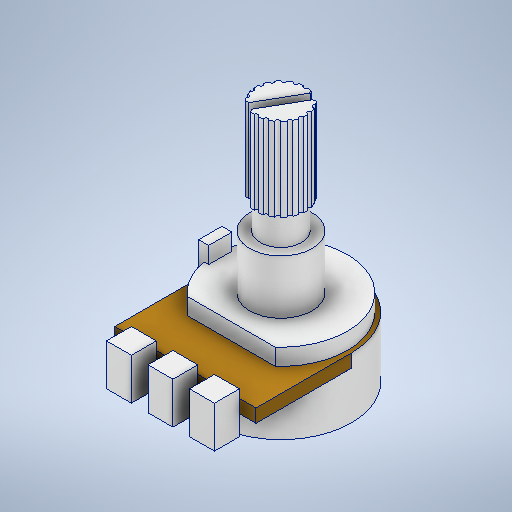
# Autodesk Inventor part: volume
Saved by Autodesk Inventor 2026.1 (Build 301233020, 233B)
## iProperties
Created: 2026-02-01
Part Number: volume
Material: アルミニウム 6061
Document SubType Name: Modeling
Designer: hibik
Density: 2.7 g/cm^3
Appearance: アルミニウム - フラット
Author: hibik
Autodesk Inventor part; units mm, degrees
ref_plane "YZ Plane" through (0, 0, 0) normal (1, 0, 0) x (0, 1, 0)
ref_plane "XZ Plane" through (0, 0, 0) normal (0, 1, 0) x (-1, 0, 0)
ref_plane "XY Plane" through (0, 0, 0) normal (0, 0, 1) x (1, 0, 0)
sketch "スケッチ1" plane through (0, 0, 0) normal (0, 1, 0) x (-1, 0, 0)
  circle A0 centre (0, 0) radius 8.5
  dimension "d0" = 17
  constraints: 1 centre point, 1 coincident
  measures "d0" diameter of A0
extrude "押し出し1" add sketch "スケッチ1" along normal blind 9.3
sketch "スケッチ2" plane through (0, 9.3, 0) normal (0, 1, 0) x (1, 0, 0)
  circle A0 centre (0, 0) radius 3
  dimension "d3" = 6
  constraints: 1 centre point, 1 coincident
  measures "d3" diameter of A0
extrude "押し出し2" add sketch "スケッチ2" along normal blind 20
sketch "スケッチ3" plane through (0, 9.3, 0) normal (0, 1, 0) x (1, 0, 0)
  circle A0 centre (0, 0) radius 3.75
  dimension "d6" = 7.5
  constraints: 1 centre point, 1 coincident
  measures "d6" diameter of A0
extrude "押し出し3" add sketch "スケッチ3" along normal blind 6.5
sketch "スケッチ4" plane through (0, 15.8, 0) normal (0, 1, 0) x (1, 0, 0)
  circle A0 centre (0, 0) radius 3 projected
  circle A1 centre (0, 0) radius 2.5
  dimension "d9" = 5
  constraints: 1 centre point, 1 coincident
  measures "d9" diameter of A1
extrude "押し出し4" cut sketch "スケッチ4" along normal blind 3.5
sketch "スケッチ5" plane through (0, 9.3, 0) normal (0, 1, 0) x (1, 0, 0)
  circle A0 centre (0, 0) radius 6
  circle A1 centre (0, 0) radius 8.5 projected
  dimension "d12" = 12
  constraints: 1 centre point, 1 coincident
  measures "d12" diameter of A0
extrude "押し出し5" cut sketch "スケッチ5" against normal blind 2
sketch "スケッチ6" plane through (0, 7.3, 0) normal (0, 1, 0) x (1, 0, 0)
  circle A0 centre (0, 0) radius 8.5 projected
  line L0 (-8.5, 0) -> (8.5, 0)
  line L1 (8.5, 0) -> (8.5, -11.5)
  line L2 (8.5, -11.5) -> (-8.5, -11.5)
  line L3 (-8.5, -11.5) -> (-8.5, 0)
  dimension "d15" = 11.5
  constraints: 8 end point, 2 parallel, 2 vertical, 1 horizontal, 1 perpendicular, 2 other
  measures "d15" distance of L2.end L0.start
extrude "押し出し6" add sketch "スケッチ6" against normal blind 1.6 contours L1 L2 L3 A0
sketch "スケッチ7" plane through (-8.5, 7.3, 11.5) normal (0, 0, 1) x (1, 0, 0)
  line L0 (7, 1) -> (10, 1)
  line L1 (10, 1) -> (10, -4)
  line L2 (10, -4) -> (7, -4)
  line L3 (7, -4) -> (7, 1)
  line L4 (0, 0) -> (17, 0) projected
  point P0 (8.5, -7.3)
  point P1 (8.5, -4)
  point P2 (8.5, 1)
  dimension "d18" = 5
  dimension "d19" = 3
  dimension "d20" = 1
  constraints: 8 end point, 2 midpoint, 2 parallel, 1 horizontal, 1 perpendicular, 1 vertical alignment
  measures "d18" distance of L0.end L1.end
  measures "d19" distance of L1.end L2.end
  measures "d20" distance from line of L4 point (8.5, 1)
extrude "押し出し7" add sketch "スケッチ7" along normal blind 3
pattern_linear "矩形状パターン1" count 2 spacing 5 along (1, 0, 0) count 2 spacing 5 along (-1, 0, 0) of "押し出し7"
sketch "スケッチ8" plane through (0, 7.3, 0) normal (0, 1, 0) x (1, 0, 0)
  line L0 (-8.5, -1.4) -> (-7.3, -1.4)
  line L1 (-7.3, -1.4) -> (-7.3, 1.4)
  line L2 (-7.3, 1.4) -> (-8.5, 1.4)
  line L3 (-8.5, 1.4) -> (-8.5, -1.4)
  point P0 (0, 0)
  point P1 (-8.5, 0)
  point P2 (-8.5, 0)
  dimension "d29" = 2.8
  dimension "d30" = 1.2
  constraints: 8 end point, 2 parallel, 1 coincident, 1 horizontal, 1 midpoint, 1 perpendicular
  measures "d29" distance of L2.end L0.start
  measures "d30" distance of L1.end L2.end
extrude "押し出し8" add sketch "スケッチ8" along normal blind 4
sketch "スケッチ9" plane through (0, 7.3, 0) normal (0, 1, 0) x (1, 0, 0)
  circle A0 centre (0, 0) radius 8
  line L0 (-5.2915, -6) -> (5.2915, -6)
  circle A1 centre (0, 0) radius 6 projected
  point P0 (0, -6)
  dimension "d33" = 16
  constraints: 2 end point, 2 point on circle, 1 centre point, 1 coincident, 1 horizontal, 1 tangent
  measures "d33" diameter of A0
extrude "押し出し9" add sketch "スケッチ9" along normal blind 2 contours A0 L0 picked at (7.1897, 1.149)
sketch "スケッチ10" plane through (0, 29.3, 0) normal (0, 1, 0) x (1, 0, 0)
  line L0 (-2.308, -2.9976) -> (-1.442, -3.4976)
  line L1 (-1.442, -3.4976) -> (2.308, 2.9976)
  line L2 (2.308, 2.9976) -> (1.442, 3.4976)
  line L3 (1.442, 3.4976) -> (-2.308, -2.9976)
  line L4 (-1.875, -3.2476) -> (1.875, 3.2476)
  line L5 (0, 20.6367) -> (0, -20.3561) construction
  circle A0 centre (0, 0) radius 3.75 projected
  point P0 (2.2913, 2.9686)
  point P1 (1.4252, 3.4686)
  point P2 (-2.2913, -2.9686)
  point P3 (-1.4252, -3.4686)
  dimension "d36" = 30
  dimension "d37" = 1
  constraints: 10 end point, 3 midpoint, 2 parallel, 1 perpendicular, 1 tangent
  measures "d36" angle of L5 L4
  measures "d37" distance between parallel lines of L1 L3
extrude "押し出し10" cut sketch "スケッチ10" against normal up to surface (10 mm away) contours A0 L3 L4 | L4 A0 L1
sketch "スケッチ11" plane through (0, 29.3, 0) normal (0, 1, 0) x (1, 0, 0)
  arc A0 (1.046, 2.8117) -> (-1.912, -2.3117) centre (0, 0) ccw projected
  circle A1 centre (0, 3) radius 0.25
  dimension "d40" = 0.5
  constraints: 1 centre point, 1 point on circle, 1 vertical alignment
  measures "d40" diameter of A1
extrude "押し出し11" cut sketch "スケッチ11" against normal up to surface (10 mm away)
pattern_circular "円形状パターン1" count 18 over 360 about axis through (0, -10, 0) along (0, 1, 0) of "押し出し11"
